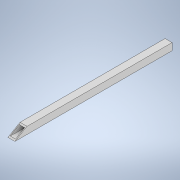
# Autodesk Inventor part: baseAluminumExtrusion
Saved by Autodesk Inventor 2020.2 (Build 242310000, 310)
## iProperties
Created: 2020-01-19
Part Number: baseAluminumExtrusion
Material: Generic
Document SubType Name: Modeling
Designer: robst
Density: 1 g/cm^3
Appearance: Default
Author: robst
Autodesk Inventor part; units mm, degrees
ref_plane "YZ Plane" through (0, 0, 0) normal (1, 0, 0) x (0, 1, 0)
ref_plane "XZ Plane" through (0, 0, 0) normal (0, 1, 0) x (-1, 0, 0)
ref_plane "XY Plane" through (0, 0, 0) normal (0, 0, 1) x (1, 0, 0)
sketch "Sketch1" plane through (0, 0, 0) normal (0, 0, 1) x (1, 0, 0)
  line L0 (-12.7, -12.7) -> (12.7, -12.7)
  line L1 (12.7, -12.7) -> (12.7, 12.7)
  line L2 (12.7, 12.7) -> (-12.7, 12.7)
  line L3 (-12.7, 12.7) -> (-12.7, -12.7)
  line L4 (-12.7, -12.7) -> (12.7, 12.7) construction
  line L5 (12.7, -12.7) -> (-12.7, 12.7) construction
  line L6 (-9.525, -9.525) -> (9.525, -9.525)
  line L7 (9.525, -9.525) -> (9.525, 9.525)
  line L8 (9.525, 9.525) -> (-9.525, 9.525)
  line L9 (-9.525, 9.525) -> (-9.525, -9.525)
  line L10 (-9.525, -9.525) -> (9.525, 9.525) construction
  line L11 (9.525, -9.525) -> (-9.525, 9.525) construction
  point P0 (0, 0)
  dimension "d0" = 25.4
  dimension "d1" = 25.4
  dimension "d2" = 3.175
  constraints: 24 end point, 4 midpoint, 4 parallel, 3 perpendicular, 2 horizontal
  measures "d0" distance of L0.start L0.end
  measures "d1" distance of L1.end L0.end
  measures "d2" distance between parallel lines of L6 L0
extrude "Extrusion1" add sketch "Sketch1" along normal mid plane 568.325
sketch "Sketch2" plane through (12.7, -12.7, 284.1625) normal (1, 0, 0) x (0, 0, -1)
  line L0 (0, 0) -> (568.325, 0) projected
  line L1 (0, 0) -> (43.9941, 25.4)
  line L2 (568.325, 25.4) -> (0, 25.4) projected
  line L3 (43.9941, 25.4) -> (0, 25.4)
  line L4 (0, 25.4) -> (0, 0)
  line L5 (0, 3.175) -> (568.325, 3.175) projected
  point P0 (284.1625, 12.7)
  dimension "d5" = 30
  constraints: 6 end point, 1 collinear, 1 perpendicular, 1 point on line
  measures "d5" angle of L1 L0
extrude "Extrusion2" cut sketch "Sketch2" against normal through all
body "Solid1"
